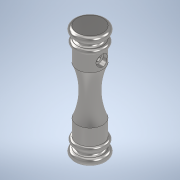
# Autodesk Inventor part: Wheel Shaft Pillar - 2
Saved by Autodesk Inventor 2021.1 (Build 251245010, 245A)
## iProperties
Created: 2025-09-17
Part Number: Wheel Shaft Pillar - 2
Material: Stainless Steel
Document SubType Name: Modeling
Designer: SD
Density: 8 g/cm^3
Appearance: Semi-Polished
Mass: 91.1348 g
Surface Area: 47.9589 cm^2
Volume: 11.3919 cm^3
Project: Automatic Tea Steeping mechanism
BOM-Mass: 0.09113
BOM-Area: 0.005
Length: 70.000 mm
Diameter: 20.000 mm
Author: SD
Title: Wheel Shaft Pillar - 2
Autodesk Inventor part; units mm, degrees
ref_plane "XZ Plane" through (0, 0, 0) normal (0, 1, 0) x (-1, 0, 0)
sketch "Sketch1" plane through (0, 0, 0) normal (0, 0, 1) x (1, 0, 0)
  line L0 (0, 0) -> (0, -70)
  line L1 (0, 0) -> (8, 0)
  line L2 (8, 0) -> (8, -4) construction
  arc A0 (8, -4) -> (8, 0) centre (8, -2) ccw
  arc A1 (8, -4) -> (8, -7) centre (8, -5.5) ccw
  line L3 (8, -5.5) -> (4.7369, -5.5) construction
  arc A2 (8, -10) -> (8, -7) centre (8, -8.5) ccw
  line L4 (0, -70) -> (8, -70)
  line L5 (8, -70) -> (8, -66) construction
  arc A3 (8, -70) -> (8, -66) centre (8, -68) ccw
  arc A4 (8, -63) -> (8, -66) centre (8, -64.5) ccw
  arc A5 (8, -63) -> (8, -60) centre (8, -61.5) ccw
  arc A6 (8, -20) -> (8, -50) centre (45.081, -35) ccw
  line L6 (8, -10) -> (8, -20)
  line L7 (8, -50) -> (8, -60)
  dimension "d1" = 10
  dimension "d2" = 4
  dimension "d3" = 1.5
  dimension "d4" = 3
  dimension "d5" = 3
  dimension "d6" = 1.5
  dimension "d7" = 4
  dimension "d8" = 10
  dimension "d9" = 1.5
  dimension "d10" = 3
  dimension "d11" = 3
  dimension "d12" = 1.5
  dimension "d16" = 20
  dimension "d17" = 20
  dimension "d18" = 40
  dimension "d19" = 10
  dimension "d20" = 10
  constraints: 16 end point, 14 point on circle, 7 centre point, 5 vertical alignment, 3 horizontal, 3 vertical, 2 midpoint
  measures "d2" distance of L1.end L2.end
  measures "d3" radius of A1
  measures "d4" distance of A1.end L2.end
  measures "d5" distance of A1.end L6.start
  measures "d6" radius of A2
  measures "d7" distance of L4.end L5.end
  measures "d9" radius of A4
  measures "d10" distance of L5.end A4.start
  measures "d11" distance of A4.start L7.end
  measures "d12" radius of A5
  measures "d16" distance from line of L6.end L1
  measures "d17" distance from line of L7.start L4
  measures "d18" radius of A6
  measures "d19" distance of L6.start L6.end
  measures "d20" distance of L7.start L7.end
revolve "Revolution1" add sketch "Sketch1" angle 360 about axis through (0, 0, 0) along (0, -1, 0)
ref_plane "Work Plane1" through (8, 0, 0) normal (1, 0, 0) x (0, 1, 0)
sketch "Sketch3" plane through (8, 0, 0) normal (1, 0, 0) x (0, 1, 0)
  circle A0 centre (-15, 0) radius 3.5
  line L0 (-70, 8) -> (-70, -8) projected
  point P0 (0, 0)
  dimension "d24" = 7
  dimension "d25" = 55
  constraints: 1 centre point, 1 horizontal alignment
  measures "d24" diameter of A0
  measures "d25" distance from line of L0 A0.centre
extrude "Extrusion2" cut sketch "Sketch3" against normal blind 3
ref_plane "Work Plane2" through (-8, 0, 0) normal (1, 0, 0) x (0, 1, 0)
sketch "Sketch5" plane through (0, -70, 0) normal (0, -1, 0) x (1, 0, 0)
  point P0 (0, 0)
  point P1 (0, 0)
  constraints: 1 coincident
hole "Hole1" at (0, -70, 0) direction (0, 1, 0) diameter 6.647 depth 22.2 tip angle 118 thread size "M8x1.25" class "6H" standard "ISO Metric profile"
sketch "Sketch6" plane through (5, -15, 0) normal (1, 0, 0) x (0, 0, -1)
  circle A0 centre (0, 0) radius 2
  line L0 (-8, -55) -> (8, -55) projected
  point P0 (0, 15)
  point P1 (0, 3.5)
  point P2 (0, -3.5)
  dimension "d39" = 4
  dimension "d40" = 55
  constraints: 3 vertical alignment, 1 centre point
  measures "d39" diameter of A0
  measures "d40" distance from line of L0 A0.centre
extrude "Extrusion4" cut sketch "Sketch6" against normal blind 1
body "Solid1"
